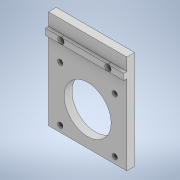
# Autodesk Inventor part: motor mount lower
Saved by Autodesk Inventor 2021 (Build 250183000, 183)
## iProperties
Created: 2022-09-08
Part Number: motor mount lower
Material: Generic
Document SubType Name: Modeling
Designer: szucs
Density: 1 g/cm^3
Appearance: Default
Author: szucs
Autodesk Inventor part; units mm, degrees
ref_plane "YZ Plane" through (0, 0, 0) normal (1, 0, 0) x (0, 1, 0)
ref_plane "XZ Plane" through (0, 0, 0) normal (0, 1, 0) x (-1, 0, 0)
ref_plane "XY Plane" through (0, 0, 0) normal (0, 0, 1) x (1, 0, 0)
sketch "Sketch1" plane through (0, 0, 0) normal (0, 0, 1) x (1, 0, 0)
  line L0 (0, 88.2) -> (0, -88.2) projected
  line L1 (-70, 0) -> (70, 0) projected
  line L2 (-50, -63) -> (50, -63)
  line L3 (50, -63) -> (50, 63)
  line L4 (50, 63) -> (-50, 63)
  line L5 (-50, 63) -> (-50, -63)
  circle A0 centre (0, -20) radius 30
  circle A1 centre (-30, 43) radius 4
  circle A2 centre (30, 43) radius 4
  circle A3 centre (34.8, -54.8) radius 3.25
  circle A4 centre (34.8, 14.8) radius 3.25
  circle A5 centre (-34.8, 14.8) radius 3.25
  circle A6 centre (-34.8, -54.8) radius 3.25
  line L6 (-30, 43) -> (-30, 39)
  line L7 (0, -20) -> (0, 10)
  point P0 (0, 0)
  dimension "d2" = 60
  dimension "d4" = 8
  dimension "d0" = 100
  dimension "d1" = 126
  dimension "d3" = 43
  dimension "d5" = 8
  dimension "d6" = 20
  dimension "d7" = 20
  dimension "d8" = 20
  dimension "d9" = 20
  dimension "d10" = 6.5
  dimension "d11" = 6.5
  dimension "d12" = 6.5
  dimension "d13" = 6.5
  dimension "d14" = 69.6
  dimension "d15" = 69.6
  dimension "d16" = 69.6
  dimension "d17" = 69.6
  dimension "d18" = 0
  dimension "d19" = 0
  dimension "d20" = 34.8
  dimension "d21" = 34.8
  dimension "d22" = 29
  constraints: 12 end point, 5 centre point, 2 parallel, 2 point on line, 2 vertical alignment, 1 horizontal, 1 perpendicular, 1 vertical, 6 other
  measures "d0" distance of L4.end L3.end
  measures "d1" distance of L3.end L2.end
  measures "d3" distance from line of L2 L7.start
  measures "d5" diameter of A2
  measures "d6" distance from line of L4 L6.start
  measures "d7" distance from line of L5 L6.start
  measures "d8" distance from line of L3 A2.centre
  measures "d9" distance from line of L4 A2.centre
  measures "d10" diameter of A3
  measures "d11" diameter of A4
  measures "d12" diameter of A5
  measures "d13" diameter of A6
  measures "d14" distance of A5.centre A6.centre
  measures "d15" distance of A3.centre A4.centre
  measures "d16" distance of A6.centre A3.centre
  measures "d17" distance of A5.centre A4.centre
  measures "d18" vertical distance of A4.centre A5.centre
  measures "d19" horizontal distance of A5.centre A6.centre
  measures "d20" distance from line of L0 A5.centre
  measures "d21" horizontal distance of A5.centre L7.start
  measures "d22" vertical distance of L7.end L6.end
extrude "Extrusion1" add sketch "Sketch1" along normal blind 20 contours L4 L3 L1 A0 L0 | L0 A0 L1 L5 L4 | L1 L3 L2 L0 A0 | A0 L0 L2 L5 L1
sketch "Sketch2" plane through (0, 0, 20) normal (0, 0, 1) x (1, 0, 0)
  line L0 (50, 63) -> (-50, 63) projected
  line L1 (-50, 63) -> (-50, -63) projected
  line L2 (-50, -63) -> (50, -63) projected
  line L3 (50, -63) -> (50, 63) projected
  circle A0 centre (30, 43) radius 4 projected
  circle A1 centre (34.8, 14.8) radius 3.25 projected
  circle A2 centre (34.8, -54.8) radius 3.25 projected
  circle A3 centre (-34.8, -54.8) radius 3.25 projected
  circle A4 centre (-34.8, 14.8) radius 3.25 projected
  circle A5 centre (-30, 43) radius 4 projected
  circle A6 centre (0, -20) radius 30 projected
  line L4 (-50, 63) -> (-50, -63) projected
  line L5 (-50, 43) -> (50, 43)
  line L6 (-50, 47) -> (50, 47)
  line L7 (-50, 39) -> (50, 39)
  point P0 (0, 0)
  dimension "d25" = 4
  dimension "d26" = 4
  constraints: 6 end point, 3 point on line, 2 parallel, 1 perpendicular
  measures "d25" distance between parallel lines of L5 L6
  measures "d26" distance between parallel lines of L5 L7
extrude "Extrusion2" cut sketch "Sketch2" against normal blind 4 contours L3 L6 L1 L0 | L3 L2 L1 L7
sketch "Sketch3" plane through (0, 0, 0) normal (0, 0, -1) x (-1, 0, 0)
  line L0 (-50, 63) -> (50, 63) projected
  line L1 (-50, -63) -> (-50, 63) projected
  line L2 (50, -63) -> (-50, -63) projected
  line L3 (50, 63) -> (50, -63) projected
  circle A0 centre (-30, 43) radius 4 projected
  circle A1 centre (-34.8, 14.8) radius 3.25 projected
  circle A2 centre (-34.8, -54.8) radius 3.25 projected
  circle A3 centre (34.8, -54.8) radius 3.25 projected
  circle A4 centre (34.8, 14.8) radius 3.25 projected
  circle A5 centre (30, 43) radius 4 projected
  circle A6 centre (0, -20) radius 30 projected
  point P0 (0, 0)
extrude "Extrusion3" cut sketch "Sketch3" against normal blind 6
body "Solid1"
